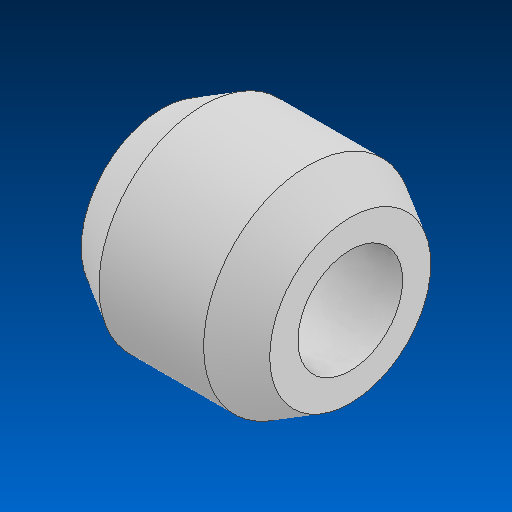
# Autodesk Inventor part: hudson1-37
Saved by Autodesk Inventor 2025.2 (Build 292293000, 293)
## iProperties
Created: 2024-11-07
Part Number: hudson1-37
Material: Genérico
Document SubType Name: Modeling
Designer: Steven C
Density: 1 g/cm^3
Appearance: Valor por defecto
Sending System: Autodesk Inventor 2025
Preprocessor: ST-DEVELOPER v20
Title: hudson1-37.stp
Author: Steven C
Autodesk Inventor part; units mm, degrees
ref_plane "YZ Plane" through (0, 0, 0) normal (1, 0, 0) x (0, 1, 0)
ref_plane "XZ Plane" through (0, 0, 0) normal (0, 1, 0) x (-1, 0, 0)
ref_plane "XY Plane" through (0, 0, 0) normal (0, 0, 1) x (1, 0, 0)
sketch "Boceto1" plane through (0, 0, 0) normal (0, 0, 1) x (1, 0, 0)
  line L0 (0, 0) -> (9, 0)
  line L1 (9, 0) -> (9, 5)
  line L2 (9, 5) -> (0, 5)
  line L3 (0, 5) -> (0, 0)
  line L4 (-11.6146, 0) -> (11.6146, 0)
  line L5 (0, 0) -> (0, 2.5)
  line L6 (0, 2.5) -> (2.5247, -1.873)
  dimension "d0" = 9
  dimension "d1" = 5
  dimension "d3" = 2.5
  dimension "d4" = 5
  dimension "d5" = 30
  constraints: 14 end point, 2 horizontal, 2 midpoint, 2 parallel, 1 perpendicular
  measures "d0" distance of L2.end L1.end
  measures "d1" distance of L0.end L1.end
  measures "d3" distance of L0.start L5.end
  measures "d4" distance of L2.end L0.start
  measures "d5" angle of L6 L3
revolve "Revolución1" add sketch "Boceto1" angle 360 about axis through (-11.6146, 0, 0) along (1, 0, 0)
chamfer "Chaflán1" distance 2 angle 30 2 edges at (0, -5, 0) (9, -5, 0) measured on face at (6, 4.9838, -0.4023)
sketch "Boceto2" plane through (9, 0, 0) normal (1, 0, 0) x (0, 0, -1)
  circle A0 centre (0, 0) radius 5 projected
  point P0 (0, 0)
  constraints: 1 coincident
hole "Agujero1" at (9, 0, 0) direction (-1, 0, 0) diameter 5 end through all
